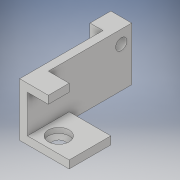
# Autodesk Inventor part: WheelIntake4.0Base
Saved by Autodesk Inventor 2017 (Build 210142000, 142)
## iProperties
Created: 2017-12-13
Part Number: WheelIntake4.0Base
Material: Generic
Document SubType Name: Modeling
Designer: User
Density: 1 g/cm^3
Appearance: Default
Author: User
Autodesk Inventor part; units mm, degrees
ref_plane "YZ Plane" through (0, 0, 0) normal (1, 0, 0) x (0, 1, 0)
ref_plane "XZ Plane" through (0, 0, 0) normal (0, 1, 0) x (-1, 0, 0)
ref_plane "XY Plane" through (0, 0, 0) normal (0, 0, 1) x (1, 0, 0)
sketch "Sketch1" plane through (0, 0, 0) normal (1, 0, 0) x (0, 1, 0)
  line L0 (0, 0) -> (32.5438, 0)
  line L1 (32.5438, 0) -> (32.5438, -63.5)
  line L2 (32.5438, -63.5) -> (0, -63.5)
  line L3 (0, -63.5) -> (0, 0)
  dimension "d0" = 32.5438
  dimension "d1" = 63.5
  constraints: 8 end point, 2 parallel, 1 horizontal, 1 perpendicular
  measures "d0" distance of L1.end L2.end
  measures "d1" distance of L0.end L1.end
extrude "Extrusion1" add sketch "Sketch1" along normal blind 4.7625
sketch "Sketch2" plane through (4.7625, 0, 0) normal (1, 0, 0) x (0, 0, -1)
  line L0 (0, 32.5438) -> (0, 0) projected
  line L1 (0, 0) -> (63.5, 0) projected
  line L2 (63.5, 0) -> (63.5, 32.5438) projected
  line L3 (63.5, 32.5438) -> (0, 32.5438) projected
  line L4 (0, 32.5438) -> (12.7, 32.5438)
  line L5 (12.7, 32.5438) -> (12.7, 27.7812)
  line L6 (12.7, 27.7812) -> (0, 27.7812)
  line L7 (0, 27.7812) -> (0, 32.5438)
  dimension "d4" = 12.7
  dimension "d5" = 4.7625
  constraints: 8 end point, 2 parallel, 1 horizontal, 1 perpendicular
  measures "d4" distance of L5.end L6.end
  measures "d5" distance of L4.end L5.end
extrude "Extrusion2" add sketch "Sketch2" along normal blind 12.7 contours L3 L5 L6 L0
sketch "Sketch3" plane through (4.7625, 0, 0) normal (1, 0, 0) x (0, 0, -1)
  line L0 (12.7, 27.7812) -> (0, 27.7812) projected
  line L1 (0, 27.7812) -> (0, 0) projected
  line L2 (0, 0) -> (63.5, 0) projected
  line L3 (63.5, 0) -> (63.5, 32.5438) projected
  line L4 (63.5, 32.5438) -> (12.7, 32.5438) projected
  line L5 (12.7, 32.5438) -> (12.7, 27.7812) projected
  line L6 (0, 0) -> (25.4, 0)
  line L7 (25.4, 0) -> (25.4, 4.7625)
  line L8 (25.4, 4.7625) -> (0, 4.7625)
  line L9 (0, 4.7625) -> (0, 0)
  dimension "d8" = 4.7625
  constraints: 8 end point, 2 parallel, 1 horizontal, 1 perpendicular
  measures "d8" distance of L7.end L6.end
extrude "Extrusion3" add sketch "Sketch3" along normal blind 25.4 contours L8 L7 L2 L1
sketch "Sketch4" plane through (0, 0, 0) normal (-1, 0, 0) x (0, 0, 1)
  line L0 (0, 0) -> (0, 32.5438) projected
  line L1 (0, 32.5438) -> (-63.5, 32.5438) projected
  line L2 (-63.5, 32.5438) -> (-63.5, 0) projected
  line L3 (-63.5, 0) -> (0, 0) projected
  line L4 (-63.5, 32.5438) -> (-12.7, 32.5438) projected
  line L5 (-63.5, 32.5438) -> (-50.8, 32.5438)
  line L6 (-50.8, 32.5438) -> (-50.8, 16.6688)
  line L7 (-50.8, 16.6688) -> (-63.5, 16.6688)
  line L8 (-63.5, 16.6688) -> (-63.5, 32.5438)
  dimension "d11" = 12.7
  dimension "d12" = 15.875
  constraints: 8 end point, 2 parallel, 1 horizontal, 1 perpendicular
  measures "d11" distance of L6.end L7.end
  measures "d12" distance of L5.end L6.end
extrude "Extrusion4" add sketch "Sketch4" along normal blind 7.9375 contours L2 L1 L6 L7
sketch "Sketch5" plane through (4.7625, 0, 0) normal (1, 0, 0) x (0, 0, -1)
  line L0 (25.4, 4.7625) -> (25.4, 0) projected
  line L1 (25.4, 0) -> (63.5, 0) projected
  line L2 (63.5, 0) -> (63.5, 32.5438) projected
  line L3 (63.5, 32.5438) -> (12.7, 32.5438) projected
  line L4 (12.7, 32.5438) -> (12.7, 27.7812) projected
  line L5 (12.7, 27.7812) -> (0, 27.7812) projected
  line L6 (0, 27.7812) -> (0, 4.7625) projected
  line L7 (0, 4.7625) -> (25.4, 4.7625) projected
  line L8 (0, 32.5438) -> (0, 27.7812) projected
  line L9 (0, 27.7812) -> (12.7, 27.7812) projected
  line L10 (12.7, 27.7812) -> (12.7, 32.5438) projected
  line L11 (12.7, 32.5438) -> (0, 32.5438) projected
  point P0 (0, 0)
  point P1 (57.15, 24.6063)
  dimension "d15" = 4.7625
  dimension "d16" = 7.9375
  dimension "d17" = 6.35
  measures "d15" distance of L3.end L4.end
  measures "d16" distance from line of L3 point (57.15, 24.606)
  measures "d17" distance from line of L2 point (57.15, 24.606)
hole "Hole1" at (4.7625, 24.6063, -57.15) direction (-1, 0, 0) diameter 6.858 end through all
sketch "Sketch6" plane through (4.7625, 4.7625, 0) normal (0, 1, 0) x (1, 0, 0)
  line L0 (0, 0) -> (0, 25.4) projected
  line L1 (0, 0) -> (25.4, 0) projected
  line L2 (25.4, 25.4) -> (25.4, 0) projected
  line L3 (0, 25.4) -> (25.4, 25.4) projected
  point P0 (-4.7625, 0)
  point P1 (9.525, 9.525)
  dimension "d25" = 9.525
  dimension "d26" = 9.525
  measures "d25" distance from line of L0 point (9.525, 9.525)
  measures "d26" distance from line of L1 point (9.525, 9.525)
hole "Hole2" at (14.2875, 4.7625, -9.525) direction (0, -1, 0) diameter 12.7 depth 3.175 tip angle 118
body "Solid1"
